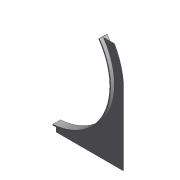
# Autodesk Inventor part: ShooterCurve
Saved by Autodesk Inventor 2012 (Build 160160000, 160)
## iProperties
Created: 2012-01-27
Part Number: ShooterCurve
Material: Aluminum-6061
Document SubType Name: Modeling
Designer: JesseK
Mass: 472.226 g
Surface Area: 1431.15 cm^2
Volume: 174.253 cm^3
Density: 2.71 g/cm^3
Author: JesseK
Autodesk Inventor part; units mm, degrees
ref_plane "YZ Plane" through (0, 0, 0) normal (1, 0, 0) x (0, 1, 0)
ref_plane "XZ Plane" through (0, 0, 0) normal (0, 1, 0) x (-1, 0, 0)
ref_plane "XY Plane" through (0, 0, 0) normal (0, 0, 1) x (1, 0, 0)
sketch "Sketch1" plane through (0, 0, 0) normal (0, 0, 1) x (1, 0, 0)
  line L0 (-168.2745, 480.6024) -> (-113.8232, 480.6024)
  line L1 (-73.2956, 353.1342) -> (-73.2956, 2.8452)
  line L2 (-73.2956, 2.8452) -> (-375.9641, 2.8452)
  line L3 (-375.9641, 2.8452) -> (-375.9641, 41.7492)
  arc A0 (-375.9641, 41.7492) -> (-168.2745, 480.6024) centre (-397.1456, 320.3452) ccw
  line L4 (-168.2745, 480.6024) -> (-245.12, 590.3492) construction
  line L5 (-245.12, 590.3492) -> (-245.12, 480.6024) construction
  line L6 (-245.12, 480.6024) -> (-168.2745, 480.6024) construction
  line L7 (-117.7456, 320.3452) -> (-117.7456, 124.3972) construction
  line L8 (-397.1456, 40.9452) -> (-554.9899, 40.9452) construction
  arc A1 (-73.2956, 353.1342) -> (-113.8232, 480.6024) centre (-397.1456, 320.3452) ccw
  dimension "d4" = 279.4
  dimension "d6" = 55
  dimension "d17" = 44.45
  dimension "d22" = 38.1
  constraints: 18 end point, 6 point on circle, 4 horizontal, 4 vertical, 3 tangent, 2 centre point, 1 coincident, 1 other
  measures "d4" radius of A0
  measures "d6" angle of L4 L6
  measures "d17" distance between parallel lines of L1 L7
  measures "d22" distance from line of L1.end L8
extrude "Extrusion1" add sketch "Sketch1" along normal blind 1.5875
sketch "Sketch2" plane through (0, 0, 1.5875) normal (0, 0, 1) x (1, 0, 0)
  arc A0 (-375.9641, 41.7492) -> (-168.2745, 480.6024) centre (-397.1456, 320.3452) ccw projected
  arc A1 (-375.9641, 41.7492) -> (-168.2745, 480.6024) centre (-397.1456, 320.3452) ccw
  arc A2 (-375.603, 37.0004) -> (-164.3733, 483.3341) centre (-397.1456, 320.3452) ccw
  line L0 (-397.1456, 320.3452) -> (-164.3733, 483.3341)
  line L1 (-168.2745, 480.6024) -> (-164.3733, 483.3341)
  line L2 (-397.1456, 320.3452) -> (-375.603, 37.0004)
  line L3 (-375.603, 37.0004) -> (-375.9641, 41.7492)
  point P0 (0, 0)
  dimension "d21" = 4.7625
  constraints: 8 end point, 4 point on circle, 2 centre point, 2 collinear, 1 coincident, 1 concentric
  measures "d21" radial gap between concentric circles of A2 A0
extrude "Extrusion2" add sketch "Sketch2" along normal blind 15.875 and the other way blind 19.05 contours A0 L0 A2 L2
fillet "Fillet1" radius 25.4 1 edges at (-113.8232, 480.6024, 0.7937)
body "Solid1"
